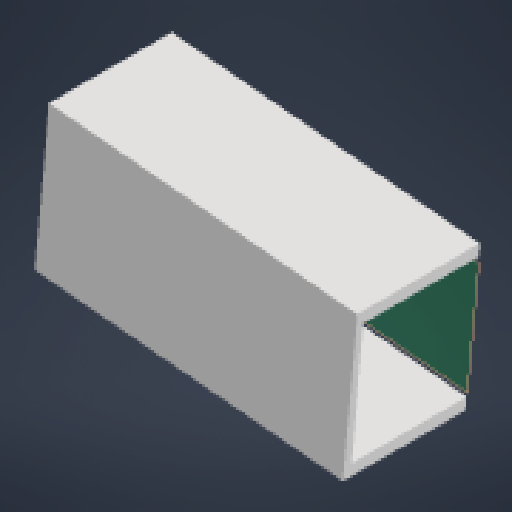
# Autodesk Inventor part: Battery_Holder
Saved by Autodesk Inventor 2024.2 (Build 282272000, 272)
## iProperties
Created: 2024-03-31
Part Number: Battery_Holder
Material: Generic
Document SubType Name: Modeling
Designer: warm
Density: 1 g/cm^3
Appearance: Default
Author: warm
Autodesk Inventor part; units mm, degrees
ref_plane "YZ Plane" through (0, 0, 0) normal (1, 0, 0) x (0, 1, 0)
ref_plane "XZ Plane" through (0, 0, 0) normal (0, 1, 0) x (-1, 0, 0)
ref_plane "XY Plane" through (0, 0, 0) normal (0, 0, 1) x (1, 0, 0)
ref_plane "Work Plane1" through (-774.147, 14.6804, 0) normal (0, 0, -1) x (0.5974542, -0.801903, 0)
sketch "Sketch1" plane through (-774.147, 14.6804, 0) normal (0, 0, -1) x (0.5974542, -0.801903, 0)
  line L0 (58.7225, -26.2361) -> (-57.2775, -26.2361)
  line L1 (-57.2775, -26.2361) -> (-57.2775, 25.7639)
  line L2 (-57.2775, 25.7639) -> (58.7225, 25.7639)
  line L3 (58.7225, 25.7639) -> (58.7225, -26.2361)
  arc A0 (19.6988, -21.7639) -> (2.3103, -21.7639) centre (11.0046, -62.2541) ccw construction
  arc A1 (19.6988, -21.7639) -> (24.3194, -21.7639) centre (22.0091, -11.0045) ccw construction
  arc A2 (41.7079, -21.7639) -> (24.3194, -21.7639) centre (33.0137, -62.2541) ccw construction
  arc A3 (41.7079, -21.7639) -> (54.7775, -8.6943) centre (44.0182, -11.0045) ccw construction
  arc A4 (54.7775, 8.6943) -> (54.7775, -8.6943) centre (95.2678, 0) ccw construction
  arc A5 (54.7775, 8.6943) -> (41.7079, 21.7639) centre (44.0182, 11.0046) ccw construction
  arc A6 (24.3194, 21.7639) -> (41.7079, 21.7639) centre (33.0137, 62.2541) ccw construction
  arc A7 (24.3194, 21.7639) -> (19.6988, 21.7639) centre (22.0091, 11.0046) ccw construction
  arc A8 (2.3103, 21.7639) -> (19.6988, 21.7639) centre (11.0046, 62.2541) ccw construction
  arc A9 (2.3103, 21.7639) -> (-2.3103, 21.7639) centre (0, 11.0046) ccw construction
  arc A10 (-19.6988, 21.7639) -> (-2.3103, 21.7639) centre (-11.0045, 62.2541) ccw construction
  arc A11 (-19.6988, 21.7639) -> (-24.3194, 21.7639) centre (-22.0091, 11.0046) ccw construction
  arc A12 (-41.7079, 21.7639) -> (-24.3194, 21.7639) centre (-33.0136, 62.2541) ccw construction
  arc A13 (-41.7079, 21.7639) -> (-54.7775, 8.6943) centre (-44.0182, 11.0046) ccw construction
  arc A14 (-54.7775, -8.6943) -> (-54.7775, 8.6943) centre (-95.2678, 0) ccw construction
  arc A15 (-54.7775, -8.6943) -> (-41.7079, -21.7639) centre (-44.0182, -11.0045) ccw construction
  arc A16 (-24.3194, -21.7639) -> (-41.7079, -21.7639) centre (-33.0136, -62.2541) ccw construction
  arc A17 (-24.3194, -21.7639) -> (-19.6988, -21.7639) centre (-22.0091, -11.0045) ccw construction
  arc A18 (-2.3103, -21.7639) -> (-19.6988, -21.7639) centre (-11.0045, -62.2541) ccw construction
  arc A19 (-2.3103, -21.7639) -> (2.3103, -21.7639) centre (0, -11.0045) ccw construction
  line L4 (159.874, 0.748) -> (161.144, 0.748) construction
  line L5 (161.144, 0.748) -> (161.144, -3.697) construction
  line L6 (159.874, -3.697) -> (161.144, -3.697) construction
  line L7 (159.874, -3.697) -> (159.874, 0.748) construction
  line L8 (63.7225, -31.2361) -> (-62.2775, -31.2361)
  line L9 (-62.2775, -31.2361) -> (-62.2775, 30.7639)
  line L10 (-62.2775, 30.7639) -> (63.7225, 30.7639)
  line L11 (63.7225, 30.7639) -> (63.7225, -31.2361)
  line L12 (58.7225, -26.2361) -> (63.7225, -26.2361)
  line L13 (-57.2775, -26.2361) -> (-62.2775, -26.2361)
  line L14 (-57.2775, 25.7639) -> (-62.2775, 25.7639)
  line L15 (58.7225, 25.7639) -> (63.7225, 25.7639)
  point P0 (474.2897, -612.02)
  dimension "d0" = 116
  dimension "d1" = 52
  dimension "d2" = 2.5
  dimension "d3" = 4
  dimension "d4" = 5
  constraints: 40 point on circle, 32 end point, 20 centre point, 6 point on line, 4 parallel, 4 perpendicular, 3 horizontal, 2 vertical, 67 other
  measures "d0" distance of L1.end L2.end
  measures "d1" distance of L0.end L1.end
  measures "d2" distance from line of A14.start L1
  measures "d3" distance from line of A11.end L2
  measures "d4" distance between parallel lines of L3 L11
extrude "Extrusion1" add sketch "Sketch1" against normal blind 47 contours L12 L11 L8 L9 L13 L0 | L13 L9 L14 L1 | L2 L14 L9 L10 L11 L15
sketch "Sketch2" plane through (-774.147, 14.6804, 47) normal (0, 0, 1) x (0.5974542, -0.801903, 0)
  line L0 (-62.2775, -30.7639) -> (63.7225, -30.7639) projected
  line L1 (63.7225, 31.2361) -> (-62.2775, 31.2361) projected
  line L2 (63.7225, -30.7639) -> (-62.2775, -30.7639)
  line L3 (-62.2775, -30.7639) -> (-62.2775, 31.2361)
  line L4 (-62.2775, 31.2361) -> (63.7225, 31.2361)
  line L5 (63.7225, 31.2361) -> (63.7225, -30.7639)
  point P0 (474.2897, 612.02)
  point P1 (-62.2775, -30.7639)
  point P2 (63.7225, 31.2361)
  constraints: 8 end point, 2 parallel, 1 horizontal, 1 perpendicular
extrude "Extrusion2" add sketch "Sketch2" along normal blind 3
fillet "Fillet1" radius 1.5875 6 edges at (-711.0274, -17.7567, 25) (-786.3067, 83.283, 25) (-760.7454, -54.7989, 25) (-756.7359, -51.8116, 23.5) (-715.037, -20.744, 23.5) (-836.0247, 46.2409, 25)
body "Solid1"
